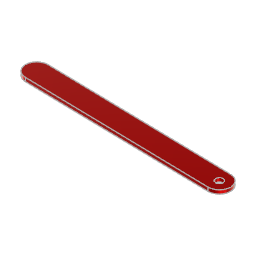
final (Autodesk Fusion 360 archive; units mm, degrees)
design "Leg"
Autodesk Fusion 360 part; units mm, degrees
sketch "Sketch1" plane through (0, 0, 0) normal (0, 0, 1) x (1, 0, 0)
  line L0 (-64.0556, -47.9598) -> (-64.1923, -47.777)
  line L1 (-64.0556, -47.9598) -> (-63.9189, -48.1426)
  arc A0 (-64.1923, -47.777) -> (-57.1589, -48.7607) centre (-60.188, -44.7827) ccw
  arc A1 (-62.8738, -41.1181) -> (-63.9189, -48.1426) centre (-59.9146, -45.1483) ccw
  line L2 (-49.93, 3.9993) -> (0.06, 2.9994)
  line L3 (-0.06, -2.9994) -> (-50.05, -1.9996)
  arc A2 (-49.93, 3.9993) -> (-50.05, -1.9996) centre (-49.99, 0.9998) ccw
  arc A3 (-0.06, -2.9994) -> (0.06, 2.9994) centre (0, 0) ccw
  circle A4 centre (0, 0) radius 1
  point P0 (-4, 4.6)
  dimension "d2" = 5
  dimension "d3" = 5
  dimension "d10" = 6
  dimension "d11" = 6
  dimension "d13" = 50
  dimension "d14" = 2
  constraint tangent L0 A0
  constraint tangent L1 A1
  constraint coincident A3.centre A4.centre
  constraint tangent L2 A3
  constraint tangent L3 A2
  constraint concentric A3 A4
  constraint tangent L2 A2
  constraint tangent L3 A3
  measures "d2" radius of A0
  measures "d3" radius of A1
  measures "d10" diameter of A3
  measures "d11" diameter of A2
  measures "d13" distance of A3.centre A2.centre
  measures "d14" diameter of A4
extrude "Extrude2" add sketch "Sketch1" along normal blind 1 contours L2 L3 A2 A3
